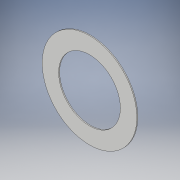
# Autodesk Inventor part: PrimaryTab
Saved by Autodesk Inventor 2019 (Build 230136000, 136)
## iProperties
Created: 2021-01-17
Part Number: PrimaryTab
Material: Типовые
Document SubType Name: Modeling
Designer: Dazer
Density: 1 g/cm^3
Appearance: По умолчанию
Author: Dazer
## iProperties of the stored document PrimaryTab_3DПЕЧАТЬ.ipt
Created: 2021-01-18
Part Number: PrimaryTab_3DПЕЧАТЬ
Material: Типовые
Document SubType Name: Modeling
Designer: Dazer
Density: 1 g/cm^3
Appearance: По умолчанию
Author: Dazer
Autodesk Inventor part; units mm, degrees
ref_plane "YZ Plane" through (0, 0, 0) normal (1, 0, 0) x (0, 1, 0)
ref_plane "XZ Plane" through (0, 0, 0) normal (0, 1, 0) x (-1, 0, 0)
ref_plane "XY Plane" through (0, 0, 0) normal (0, 0, 1) x (1, 0, 0)
sketch "Эскиз3" plane through (0, 0, 0) normal (0, 0, 1) x (1, 0, 0)
  circle A0 centre (-46, 1.5) radius 4 projected
  circle A1 centre (-46, 1.5) radius 38 projected
  line L0 (0, 0) -> (25, 0) projected
  line L1 (25, 0) -> (25, 3) projected
  line L2 (0, 3) -> (25, 3) projected
  line L3 (0, 0) -> (0, 3) projected
  circle A2 centre (-46, 1.5) radius 70.8
  circle A3 centre (-46, 1.5) radius 46.2
  constraints: 2 centre point, 2 coincident
extrude "Выдавливание2" add sketch "Эскиз3" along normal blind 1.5 contours A3 L2 A2 L0 | L0 A2 L2 A3
